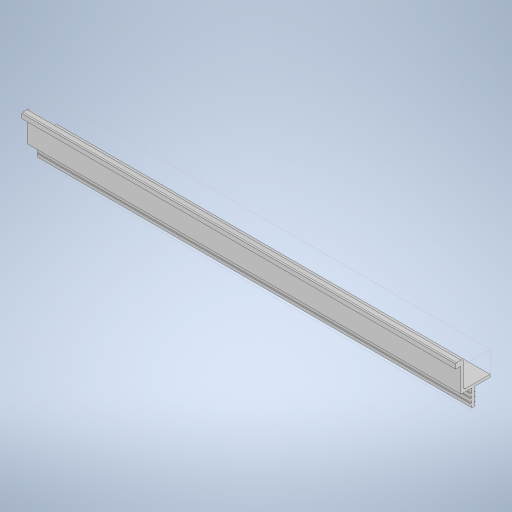
# Autodesk Inventor part: Hafele alu 126_35
Saved by Autodesk Inventor 2024 (Build 280153000, 153)
## iProperties
RuleStatus: InUse
Created: 2019-10-04
Part Number: Hafele alu 126_35
Material: Generic
Document SubType Name: Modeling
Designer: RokasM
Density: 1 g/cm^3
Appearance: Default
Author: RokasM
Autodesk Inventor part; units mm, degrees
ref_plane "YZ Plane" through (0, 0, 0) normal (1, 0, 0) x (0, 1, 0)
ref_plane "XZ Plane" through (0, 0, 0) normal (0, 1, 0) x (-1, 0, 0)
ref_plane "XY Plane" through (0, 0, 0) normal (0, 0, 1) x (1, 0, 0)
sketch "Sketch1" plane through (0, 0, 0) normal (1, 0, 0) x (0, 1, 0)
  line L0 (0, 0) -> (0, 14)
  line L1 (0, 14) -> (-3, 14)
  line L2 (-3, 14) -> (-3, 17)
  line L3 (-3, 17) -> (1.5, 17)
  line L4 (1.5, 17) -> (1.5, 1.5)
  line L5 (1.5, 1.5) -> (16.8, 1.5)
  line L6 (16.8, 1.5) -> (16.8, 0)
  line L7 (16.8, 0) -> (7.6, 0)
  line L8 (7.6, 0) -> (7.6, -2.5)
  line L9 (7.6, -2.5) -> (8.225, -2.5)
  line L10 (8.225, -2.5) -> (7.6, -5)
  line L11 (7.6, -5) -> (8.225, -5)
  line L12 (8.225, -5) -> (7.6, -7.5)
  line L13 (7.6, -7.5) -> (8.225, -7.5)
  line L14 (8.225, -7.5) -> (7.6, -10)
  line L15 (7.6, -10) -> (6.2, -10)
  line L16 (6.2, -10) -> (5.575, -7.5)
  line L17 (5.575, -7.5) -> (6.2, -7.5)
  line L18 (6.2, -7.5) -> (5.575, -5)
  line L19 (5.575, -5) -> (6.2, -5)
  line L20 (6.2, -5) -> (5.575, -2.5)
  line L21 (5.575, -2.5) -> (6.2, -2.5)
  line L22 (6.2, -2.5) -> (6.2, 0)
  line L23 (6.2, 0) -> (0, 0)
  dimension "d0" = 3
  dimension "d1" = 3
  dimension "d2" = 1.5
  dimension "d3" = 1.5
  dimension "d4" = 10
  dimension "d5" = 2.65
  dimension "d6" = 19.8
  dimension "d7" = 14
  dimension "d8" = 2.5
  dimension "d9" = 0.625
  dimension "d10" = 9.2
  constraints: 48 end point, 10 equal length, 8 horizontal, 6 vertical, 4 collinear, 2 coincident, 2 parallel, 2 vertical alignment
  measures "d0" distance between parallel lines of L1 L3
  measures "d1" distance between parallel lines of L0 L2
  measures "d2" distance between parallel lines of L4 L0
  measures "d3" distance between parallel lines of L7 L5
  measures "d4" distance between parallel lines of L15 L7
  measures "d5" distance of L13.end L16.end
  measures "d6" distance between parallel lines of L2 L6
  measures "d7" distance between parallel lines of L23 L1
  measures "d8" distance between parallel lines of L11 L13
  measures "d9" distance of L20.end L21.end
  measures "d10" distance between parallel lines of L6 L8
extrude "01_ex1" add sketch "Sketch1" along normal mid plane 250
fillet "01_fillet" radius 1.5 1 edges at (0, 1.5, 17)
fillet "01_fillet" radius 1 1 edges at (0, 1.5, 1.5)
fillet "01_fillet" radius 0.5 1 edges at (0, -3, 17)
fillet "01_fillet" radius 0.2 8 edges at (0, 8.225, -2.5) (0, 5.575, -2.5) (0, 5.575, -5) (0, 8.225, -5) (0, 8.225, -7.5) (0, 5.575, -7.5) (0, 6.2, -10) (0, 7.6, -10)
sketch "Sketch2" plane through (0, 0, 0) normal (1, 0, 0) x (0, 1, 0)
  line L0 (5.65, 0) -> (5.65, -11)
  line L1 (5.65, -11) -> (8.15, -11)
  line L2 (8.15, -11) -> (8.15, 0)
  line L3 (6.3562, -10) -> (7.4438, -10) projected
  line L4 (7.6, 0) -> (16.8, 0) projected
  line L5 (5.65, 0) -> (0, 0)
  line L6 (0, 0) -> (0, 14)
  line L7 (0, 14) -> (16.8, 14)
  line L8 (16.8, 14) -> (16.8, 0)
  line L9 (16.8, 0) -> (8.15, 0)
  line L10 (0, 0) -> (6.2, 0) projected
  line L11 (0, 14) -> (0, 0) projected
  line L12 (16.8, 0) -> (16.8, 1.5) projected
  line L13 (-3, 14) -> (0, 14) projected
  point P0 (6.9, -11)
  point P1 (6.9, -10)
  dimension "d17" = 1
  dimension "d18" = 2.5
  constraints: 16 end point, 5 collinear, 2 midpoint, 1 parallel, 1 perpendicular, 1 vertical alignment
  measures "d17" distance between parallel lines of L3 L1
  measures "d18" distance between parallel lines of L0 L2
extrude "02_ex1" add sketch "Sketch2" along normal mid plane 250 separate body
equation "\"d11\" = Length"
equation "\"d19\" = Length"
equation "\"Length\" = 250"
